Autodesk Inventor part; units mm, degrees
(part 2 of 3)
  line L477 (3.0088, -4.1422) -> (3.0088, -4.3979) construction
  spline S158 degree 3 poles (3.0088, -4.3979) (3.0088, -4.6537) (3.2161, -4.861) (3.4718, -4.861) knots 0 0 0 0 1 1 1 1
  line L478 (3.0088, -4.3979) -> (3.0088, -4.6537) construction
  line L479 (3.0088, -4.6537) -> (3.2161, -4.861) construction
  line L480 (3.2161, -4.861) -> (3.4718, -4.861) construction
  spline S159 degree 3 poles (3.4718, -4.861) (3.7274, -4.861) (3.9348, -4.6537) (3.9348, -4.3979) knots 0 0 0 0 1 1 1 1
  line L481 (3.4718, -4.861) -> (3.7274, -4.861) construction
  line L482 (3.7274, -4.861) -> (3.9348, -4.6537) construction
  line L483 (3.9348, -4.6537) -> (3.9348, -4.3979) construction
  spline S160 degree 3 poles (6.5807, -4.3979) (6.5807, -4.1422) (6.3733, -3.9349) (6.1176, -3.9349) knots 0 0 0 0 1 1 1 1
  line L484 (6.5807, -4.3979) -> (6.5807, -4.1422) construction
  line L485 (6.5807, -4.1422) -> (6.3733, -3.9349) construction
  line L486 (6.3733, -3.9349) -> (6.1176, -3.9349) construction
  spline S161 degree 3 poles (6.1176, -3.9349) (5.862, -3.9349) (5.6547, -4.1422) (5.6547, -4.3979) knots 0 0 0 0 1 1 1 1
  line L487 (6.1176, -3.9349) -> (5.862, -3.9349) construction
  line L488 (5.862, -3.9349) -> (5.6547, -4.1422) construction
  line L489 (5.6547, -4.1422) -> (5.6547, -4.3979) construction
  spline S162 degree 3 poles (5.6547, -4.3979) (5.6547, -4.6537) (5.862, -4.861) (6.1176, -4.861) knots 0 0 0 0 1 1 1 1
  line L490 (5.6547, -4.3979) -> (5.6547, -4.6537) construction
  line L491 (5.6547, -4.6537) -> (5.862, -4.861) construction
  line L492 (5.862, -4.861) -> (6.1176, -4.861) construction
  spline S163 degree 3 poles (6.1176, -4.861) (6.3733, -4.861) (6.5807, -4.6537) (6.5807, -4.3979) knots 0 0 0 0 1 1 1 1
  line L493 (6.1176, -4.861) -> (6.3733, -4.861) construction
  line L494 (6.3733, -4.861) -> (6.5807, -4.6537) construction
  line L495 (6.5807, -4.6537) -> (6.5807, -4.3979) construction
  spline S164 degree 3 poles (9.2265, -4.3979) (9.2265, -4.1422) (9.0191, -3.9349) (8.7634, -3.9349) knots 0 0 0 0 1 1 1 1
  line L496 (9.2265, -4.3979) -> (9.2265, -4.1422) construction
  line L497 (9.2265, -4.1422) -> (9.0191, -3.9349) construction
  line L498 (9.0191, -3.9349) -> (8.7634, -3.9349) construction
  spline S165 degree 3 poles (8.7634, -3.9349) (8.5078, -3.9349) (8.3005, -4.1422) (8.3005, -4.3979) knots 0 0 0 0 1 1 1 1
  line L499 (8.7634, -3.9349) -> (8.5078, -3.9349) construction
  line L500 (8.5078, -3.9349) -> (8.3005, -4.1422) construction
  line L501 (8.3005, -4.1422) -> (8.3005, -4.3979) construction
  spline S166 degree 3 poles (8.3005, -4.3979) (8.3005, -4.6537) (8.5078, -4.861) (8.7634, -4.861) knots 0 0 0 0 1 1 1 1
  line L502 (8.3005, -4.3979) -> (8.3005, -4.6537) construction
  line L503 (8.3005, -4.6537) -> (8.5078, -4.861) construction
  line L504 (8.5078, -4.861) -> (8.7634, -4.861) construction
  spline S167 degree 3 poles (8.7634, -4.861) (9.0191, -4.861) (9.2265, -4.6537) (9.2265, -4.3979) knots 0 0 0 0 1 1 1 1
  line L505 (8.7634, -4.861) -> (9.0191, -4.861) construction
  line L506 (9.0191, -4.861) -> (9.2265, -4.6537) construction
  line L507 (9.2265, -4.6537) -> (9.2265, -4.3979) construction
  spline S168 degree 3 poles (11.8723, -4.3979) (11.8723, -4.1422) (11.6649, -3.9349) (11.4092, -3.9349) knots 0 0 0 0 1 1 1 1
  line L508 (11.8723, -4.3979) -> (11.8723, -4.1422) construction
  line L509 (11.8723, -4.1422) -> (11.6649, -3.9349) construction
  line L510 (11.6649, -3.9349) -> (11.4092, -3.9349) construction
  spline S169 degree 3 poles (11.4092, -3.9349) (11.1536, -3.9349) (10.9463, -4.1422) (10.9463, -4.3979) knots 0 0 0 0 1 1 1 1
  line L511 (11.4092, -3.9349) -> (11.1536, -3.9349) construction
  line L512 (11.1536, -3.9349) -> (10.9463, -4.1422) construction
  line L513 (10.9463, -4.1422) -> (10.9463, -4.3979) construction
  spline S170 degree 3 poles (10.9463, -4.3979) (10.9463, -4.6537) (11.1536, -4.861) (11.4092, -4.861) knots 0 0 0 0 1 1 1 1
  line L514 (10.9463, -4.3979) -> (10.9463, -4.6537) construction
  line L515 (10.9463, -4.6537) -> (11.1536, -4.861) construction
  line L516 (11.1536, -4.861) -> (11.4092, -4.861) construction
  spline S171 degree 3 poles (11.4092, -4.861) (11.6649, -4.861) (11.8723, -4.6537) (11.8723, -4.3979) knots 0 0 0 0 1 1 1 1
  line L517 (11.4092, -4.861) -> (11.6649, -4.861) construction
  line L518 (11.6649, -4.861) -> (11.8723, -4.6537) construction
  line L519 (11.8723, -4.6537) -> (11.8723, -4.3979) construction
  spline S172 degree 3 poles (6.5807, 12.2708) (6.5807, 12.5264) (6.3733, 12.7338) (6.1176, 12.7338) knots 0 0 0 0 1 1 1 1
  line L520 (6.5807, 12.2708) -> (6.5807, 12.5264) construction
  line L521 (6.5807, 12.5264) -> (6.3733, 12.7338) construction
  line L522 (6.3733, 12.7338) -> (6.1176, 12.7338) construction
  spline S173 degree 3 poles (6.1176, 12.7338) (5.862, 12.7338) (5.6547, 12.5264) (5.6547, 12.2708) knots 0 0 0 0 1 1 1 1
  line L523 (6.1176, 12.7338) -> (5.862, 12.7338) construction
  line L524 (5.862, 12.7338) -> (5.6547, 12.5264) construction
  line L525 (5.6547, 12.5264) -> (5.6547, 12.2708) construction
  spline S174 degree 3 poles (5.6547, 12.2708) (5.6547, 12.0151) (5.862, 11.8077) (6.1176, 11.8077) knots 0 0 0 0 1 1 1 1
  line L526 (5.6547, 12.2708) -> (5.6547, 12.0151) construction
  line L527 (5.6547, 12.0151) -> (5.862, 11.8077) construction
  line L528 (5.862, 11.8077) -> (6.1176, 11.8077) construction
  spline S175 degree 3 poles (6.1176, 11.8077) (6.3733, 11.8077) (6.5807, 12.0151) (6.5807, 12.2708) knots 0 0 0 0 1 1 1 1
  line L529 (6.1176, 11.8077) -> (6.3733, 11.8077) construction
  line L530 (6.3733, 11.8077) -> (6.5807, 12.0151) construction
  line L531 (6.5807, 12.0151) -> (6.5807, 12.2708) construction
  spline S176 degree 3 poles (9.2265, 12.2708) (9.2265, 12.5264) (9.0191, 12.7338) (8.7634, 12.7338) knots 0 0 0 0 1 1 1 1
  line L532 (9.2265, 12.2708) -> (9.2265, 12.5264) construction
  line L533 (9.2265, 12.5264) -> (9.0191, 12.7338) construction
  line L534 (9.0191, 12.7338) -> (8.7634, 12.7338) construction
  spline S177 degree 3 poles (8.7634, 12.7338) (8.5078, 12.7338) (8.3005, 12.5264) (8.3005, 12.2708) knots 0 0 0 0 1 1 1 1
  line L535 (8.7634, 12.7338) -> (8.5078, 12.7338) construction
  line L536 (8.5078, 12.7338) -> (8.3005, 12.5264) construction
  line L537 (8.3005, 12.5264) -> (8.3005, 12.2708) construction
  spline S178 degree 3 poles (8.3005, 12.2708) (8.3005, 12.0151) (8.5078, 11.8077) (8.7634, 11.8077) knots 0 0 0 0 1 1 1 1
  line L538 (8.3005, 12.2708) -> (8.3005, 12.0151) construction
  line L539 (8.3005, 12.0151) -> (8.5078, 11.8077) construction
  line L540 (8.5078, 11.8077) -> (8.7634, 11.8077) construction
  spline S179 degree 3 poles (8.7634, 11.8077) (9.0191, 11.8077) (9.2265, 12.0151) (9.2265, 12.2708) knots 0 0 0 0 1 1 1 1
  line L541 (8.7634, 11.8077) -> (9.0191, 11.8077) construction
  line L542 (9.0191, 11.8077) -> (9.2265, 12.0151) construction
  line L543 (9.2265, 12.0151) -> (9.2265, 12.2708) construction
  spline S180 degree 3 poles (9.2265, 17.5624) (9.2265, 17.8181) (9.0191, 18.0255) (8.7634, 18.0255) knots 0 0 0 0 1 1 1 1
  line L544 (9.2265, 17.5624) -> (9.2265, 17.8181) construction
  line L545 (9.2265, 17.8181) -> (9.0191, 18.0255) construction
  line L546 (9.0191, 18.0255) -> (8.7634, 18.0255) construction
  spline S181 degree 3 poles (8.7634, 18.0255) (8.5078, 18.0255) (8.3005, 17.8181) (8.3005, 17.5624) knots 0 0 0 0 1 1 1 1
  line L547 (8.7634, 18.0255) -> (8.5078, 18.0255) construction
  line L548 (8.5078, 18.0255) -> (8.3005, 17.8181) construction
  line L549 (8.3005, 17.8181) -> (8.3005, 17.5624) construction
  spline S182 degree 3 poles (8.3005, 17.5624) (8.3005, 17.3068) (8.5078, 17.0993) (8.7634, 17.0993) knots 0 0 0 0 1 1 1 1
  line L550 (8.3005, 17.5624) -> (8.3005, 17.3068) construction
  line L551 (8.3005, 17.3068) -> (8.5078, 17.0993) construction
  line L552 (8.5078, 17.0993) -> (8.7634, 17.0993) construction
  spline S183 degree 3 poles (8.7634, 17.0993) (9.0191, 17.0993) (9.2265, 17.3068) (9.2265, 17.5624) knots 0 0 0 0 1 1 1 1
  line L553 (8.7634, 17.0993) -> (9.0191, 17.0993) construction
  line L554 (9.0191, 17.0993) -> (9.2265, 17.3068) construction
  line L555 (9.2265, 17.3068) -> (9.2265, 17.5624) construction
  spline S184 degree 3 poles (6.5807, 17.5624) (6.5807, 17.8181) (6.3733, 18.0255) (6.1176, 18.0255) knots 0 0 0 0 1 1 1 1
  line L556 (6.5807, 17.5624) -> (6.5807, 17.8181) construction
  line L557 (6.5807, 17.8181) -> (6.3733, 18.0255) construction
  line L558 (6.3733, 18.0255) -> (6.1176, 18.0255) construction
  spline S185 degree 3 poles (6.1176, 18.0255) (5.862, 18.0255) (5.6547, 17.8181) (5.6547, 17.5624) knots 0 0 0 0 1 1 1 1
  line L559 (6.1176, 18.0255) -> (5.862, 18.0255) construction
  line L560 (5.862, 18.0255) -> (5.6547, 17.8181) construction
  line L561 (5.6547, 17.8181) -> (5.6547, 17.5624) construction
  spline S186 degree 3 poles (5.6547, 17.5624) (5.6547, 17.3068) (5.862, 17.0993) (6.1176, 17.0993) knots 0 0 0 0 1 1 1 1
  line L562 (5.6547, 17.5624) -> (5.6547, 17.3068) construction
  line L563 (5.6547, 17.3068) -> (5.862, 17.0993) construction
  line L564 (5.862, 17.0993) -> (6.1176, 17.0993) construction
  spline S187 degree 3 poles (6.1176, 17.0993) (6.3733, 17.0993) (6.5807, 17.3068) (6.5807, 17.5624) knots 0 0 0 0 1 1 1 1
  line L565 (6.1176, 17.0993) -> (6.3733, 17.0993) construction
  line L566 (6.3733, 17.0993) -> (6.5807, 17.3068) construction
  line L567 (6.5807, 17.3068) -> (6.5807, 17.5624) construction
  spline S188 degree 3 poles (6.5807, 14.9166) (6.5807, 15.1723) (6.3733, 15.3797) (6.1176, 15.3797) knots 0 0 0 0 1 1 1 1
  line L568 (6.5807, 14.9166) -> (6.5807, 15.1723) construction
  line L569 (6.5807, 15.1723) -> (6.3733, 15.3797) construction
  line L570 (6.3733, 15.3797) -> (6.1176, 15.3797) construction
  spline S189 degree 3 poles (6.1176, 15.3797) (5.862, 15.3797) (5.6547, 15.1723) (5.6547, 14.9166) knots 0 0 0 0 1 1 1 1
  line L571 (6.1176, 15.3797) -> (5.862, 15.3797) construction
  line L572 (5.862, 15.3797) -> (5.6547, 15.1723) construction
  line L573 (5.6547, 15.1723) -> (5.6547, 14.9166) construction
  spline S190 degree 3 poles (5.6547, 14.9166) (5.6547, 14.661) (5.862, 14.4535) (6.1176, 14.4535) knots 0 0 0 0 1 1 1 1
  line L574 (5.6547, 14.9166) -> (5.6547, 14.661) construction
  line L575 (5.6547, 14.661) -> (5.862, 14.4535) construction
  line L576 (5.862, 14.4535) -> (6.1176, 14.4535) construction
  spline S191 degree 3 poles (6.1176, 14.4535) (6.3733, 14.4535) (6.5807, 14.661) (6.5807, 14.9166) knots 0 0 0 0 1 1 1 1
  line L577 (6.1176, 14.4535) -> (6.3733, 14.4535) construction
  line L578 (6.3733, 14.4535) -> (6.5807, 14.661) construction
  line L579 (6.5807, 14.661) -> (6.5807, 14.9166) construction
  spline S192 degree 3 poles (9.2265, 14.9166) (9.2265, 15.1723) (9.0191, 15.3797) (8.7634, 15.3797) knots 0 0 0 0 1 1 1 1
  line L580 (9.2265, 14.9166) -> (9.2265, 15.1723) construction
  line L581 (9.2265, 15.1723) -> (9.0191, 15.3797) construction
  line L582 (9.0191, 15.3797) -> (8.7634, 15.3797) construction
  spline S193 degree 3 poles (8.7634, 15.3797) (8.5078, 15.3797) (8.3005, 15.1723) (8.3005, 14.9166) knots 0 0 0 0 1 1 1 1
  line L583 (8.7634, 15.3797) -> (8.5078, 15.3797) construction
  line L584 (8.5078, 15.3797) -> (8.3005, 15.1723) construction
  line L585 (8.3005, 15.1723) -> (8.3005, 14.9166) construction
  spline S194 degree 3 poles (8.3005, 14.9166) (8.3005, 14.661) (8.5078, 14.4535) (8.7634, 14.4535) knots 0 0 0 0 1 1 1 1
  line L586 (8.3005, 14.9166) -> (8.3005, 14.661) construction
  line L587 (8.3005, 14.661) -> (8.5078, 14.4535) construction
  line L588 (8.5078, 14.4535) -> (8.7634, 14.4535) construction
  spline S195 degree 3 poles (8.7634, 14.4535) (9.0191, 14.4535) (9.2265, 14.661) (9.2265, 14.9166) knots 0 0 0 0 1 1 1 1
  line L589 (8.7634, 14.4535) -> (9.0191, 14.4535) construction
  line L590 (9.0191, 14.4535) -> (9.2265, 14.661) construction
  line L591 (9.2265, 14.661) -> (9.2265, 14.9166) construction
  spline S196 degree 3 poles (6.5807, 1.6875) (6.5807, 1.9432) (6.3733, 2.1506) (6.1176, 2.1506) knots 0 0 0 0 1 1 1 1
  line L592 (6.5807, 1.6875) -> (6.5807, 1.9432) construction
  line L593 (6.5807, 1.9432) -> (6.3733, 2.1506) construction
  line L594 (6.3733, 2.1506) -> (6.1176, 2.1506) construction
  spline S197 degree 3 poles (6.1176, 2.1506) (5.862, 2.1506) (5.6547, 1.9432) (5.6547, 1.6875) knots 0 0 0 0 1 1 1 1
  line L595 (6.1176, 2.1506) -> (5.862, 2.1506) construction
  line L596 (5.862, 2.1506) -> (5.6547, 1.9432) construction
  line L597 (5.6547, 1.9432) -> (5.6547, 1.6875) construction
  spline S198 degree 3 poles (5.6547, 1.6875) (5.6547, 1.4319) (5.862, 1.2244) (6.1176, 1.2244) knots 0 0 0 0 1 1 1 1
  line L598 (5.6547, 1.6875) -> (5.6547, 1.4319) construction
  line L599 (5.6547, 1.4319) -> (5.862, 1.2244) construction
  line L600 (5.862, 1.2244) -> (6.1176, 1.2244) construction
  spline S199 degree 3 poles (6.1176, 1.2244) (6.3733, 1.2244) (6.5807, 1.4319) (6.5807, 1.6875) knots 0 0 0 0 1 1 1 1
  line L601 (6.1176, 1.2244) -> (6.3733, 1.2244) construction
  line L602 (6.3733, 1.2244) -> (6.5807, 1.4319) construction
  line L603 (6.5807, 1.4319) -> (6.5807, 1.6875) construction
  spline S200 degree 3 poles (9.2265, 1.6875) (9.2265, 1.9432) (9.0191, 2.1506) (8.7634, 2.1506) knots 0 0 0 0 1 1 1 1
  line L604 (9.2265, 1.6875) -> (9.2265, 1.9432) construction
  line L605 (9.2265, 1.9432) -> (9.0191, 2.1506) construction
  line L606 (9.0191, 2.1506) -> (8.7634, 2.1506) construction
  spline S201 degree 3 poles (8.7634, 2.1506) (8.5078, 2.1506) (8.3005, 1.9432) (8.3005, 1.6875) knots 0 0 0 0 1 1 1 1
  line L607 (8.7634, 2.1506) -> (8.5078, 2.1506) construction
  line L608 (8.5078, 2.1506) -> (8.3005, 1.9432) construction
  line L609 (8.3005, 1.9432) -> (8.3005, 1.6875) construction
  spline S202 degree 3 poles (8.3005, 1.6875) (8.3005, 1.4319) (8.5078, 1.2244) (8.7634, 1.2244) knots 0 0 0 0 1 1 1 1
  line L610 (8.3005, 1.6875) -> (8.3005, 1.4319) construction
  line L611 (8.3005, 1.4319) -> (8.5078, 1.2244) construction
  line L612 (8.5078, 1.2244) -> (8.7634, 1.2244) construction
  spline S203 degree 3 poles (8.7634, 1.2244) (9.0191, 1.2244) (9.2265, 1.4319) (9.2265, 1.6875) knots 0 0 0 0 1 1 1 1
  line L613 (8.7634, 1.2244) -> (9.0191, 1.2244) construction
  line L614 (9.0191, 1.2244) -> (9.2265, 1.4319) construction
  line L615 (9.2265, 1.4319) -> (9.2265, 1.6875) construction
  spline S204 degree 3 poles (6.5807, 30.7915) (6.5807, 31.0472) (6.3733, 31.2546) (6.1176, 31.2546) knots 0 0 0 0 1 1 1 1
  line L616 (6.5807, 30.7915) -> (6.5807, 31.0472) construction
  line L617 (6.5807, 31.0472) -> (6.3733, 31.2546) construction
  line L618 (6.3733, 31.2546) -> (6.1176, 31.2546) construction
  spline S205 degree 3 poles (6.1176, 31.2546) (5.862, 31.2546) (5.6547, 31.0472) (5.6547, 30.7915) knots 0 0 0 0 1 1 1 1
  line L619 (6.1176, 31.2546) -> (5.862, 31.2546) construction
  line L620 (5.862, 31.2546) -> (5.6547, 31.0472) construction
  line L621 (5.6547, 31.0472) -> (5.6547, 30.7915) construction
  spline S206 degree 3 poles (5.6547, 30.7915) (5.6547, 30.5359) (5.862, 30.3284) (6.1176, 30.3284) knots 0 0 0 0 1 1 1 1
  line L622 (5.6547, 30.7915) -> (5.6547, 30.5359) construction
  line L623 (5.6547, 30.5359) -> (5.862, 30.3284) construction
  line L624 (5.862, 30.3284) -> (6.1176, 30.3284) construction
  spline S207 degree 3 poles (6.1176, 30.3284) (6.3733, 30.3284) (6.5807, 30.5359) (6.5807, 30.7915) knots 0 0 0 0 1 1 1 1
  line L625 (6.1176, 30.3284) -> (6.3733, 30.3284) construction
  line L626 (6.3733, 30.3284) -> (6.5807, 30.5359) construction
  line L627 (6.5807, 30.5359) -> (6.5807, 30.7915) construction
  spline S208 degree 3 poles (9.2265, 30.7915) (9.2265, 31.0472) (9.0191, 31.2546) (8.7634, 31.2546) knots 0 0 0 0 1 1 1 1
  line L628 (9.2265, 30.7915) -> (9.2265, 31.0472) construction
  line L629 (9.2265, 31.0472) -> (9.0191, 31.2546) construction
  line L630 (9.0191, 31.2546) -> (8.7634, 31.2546) construction
  spline S209 degree 3 poles (8.7634, 31.2546) (8.5078, 31.2546) (8.3005, 31.0472) (8.3005, 30.7915) knots 0 0 0 0 1 1 1 1
  line L631 (8.7634, 31.2546) -> (8.5078, 31.2546) construction
  line L632 (8.5078, 31.2546) -> (8.3005, 31.0472) construction
  line L633 (8.3005, 31.0472) -> (8.3005, 30.7915) construction
  spline S210 degree 3 poles (8.3005, 30.7915) (8.3005, 30.5359) (8.5078, 30.3284) (8.7634, 30.3284) knots 0 0 0 0 1 1 1 1
  line L634 (8.3005, 30.7915) -> (8.3005, 30.5359) construction
  line L635 (8.3005, 30.5359) -> (8.5078, 30.3284) construction
  line L636 (8.5078, 30.3284) -> (8.7634, 30.3284) construction
  spline S211 degree 3 poles (8.7634, 30.3284) (9.0191, 30.3284) (9.2265, 30.5359) (9.2265, 30.7915) knots 0 0 0 0 1 1 1 1
  line L637 (8.7634, 30.3284) -> (9.0191, 30.3284) construction
  line L638 (9.0191, 30.3284) -> (9.2265, 30.5359) construction
  line L639 (9.2265, 30.5359) -> (9.2265, 30.7915) construction
  spline S212 degree 3 poles (9.2265, 28.1457) (9.2265, 28.4013) (9.0191, 28.6088) (8.7634, 28.6088) knots 0 0 0 0 1 1 1 1
  line L640 (9.2265, 28.1457) -> (9.2265, 28.4013) construction
  line L641 (9.2265, 28.4013) -> (9.0191, 28.6088) construction
  line L642 (9.0191, 28.6088) -> (8.7634, 28.6088) construction
  spline S213 degree 3 poles (8.7634, 28.6088) (8.5078, 28.6088) (8.3005, 28.4013) (8.3005, 28.1457) knots 0 0 0 0 1 1 1 1
  line L643 (8.7634, 28.6088) -> (8.5078, 28.6088) construction
  line L644 (8.5078, 28.6088) -> (8.3005, 28.4013) construction
  line L645 (8.3005, 28.4013) -> (8.3005, 28.1457) construction
  spline S214 degree 3 poles (8.3005, 28.1457) (8.3005, 27.89) (8.5078, 27.6826) (8.7634, 27.6826) knots 0 0 0 0 1 1 1 1
  line L646 (8.3005, 28.1457) -> (8.3005, 27.89) construction
  line L647 (8.3005, 27.89) -> (8.5078, 27.6826) construction
  line L648 (8.5078, 27.6826) -> (8.7634, 27.6826) construction
  spline S215 degree 3 poles (8.7634, 27.6826) (9.0191, 27.6826) (9.2265, 27.89) (9.2265, 28.1457) knots 0 0 0 0 1 1 1 1
  line L649 (8.7634, 27.6826) -> (9.0191, 27.6826) construction
  line L650 (9.0191, 27.6826) -> (9.2265, 27.89) construction
  line L651 (9.2265, 27.89) -> (9.2265, 28.1457) construction
  spline S216 degree 3 poles (6.5807, 28.1457) (6.5807, 28.4013) (6.3733, 28.6088) (6.1176, 28.6088) knots 0 0 0 0 1 1 1 1
  line L652 (6.5807, 28.1457) -> (6.5807, 28.4013) construction
  line L653 (6.5807, 28.4013) -> (6.3733, 28.6088) construction
  line L654 (6.3733, 28.6088) -> (6.1176, 28.6088) construction
  spline S217 degree 3 poles (6.1176, 28.6088) (5.862, 28.6088) (5.6547, 28.4013) (5.6547, 28.1457) knots 0 0 0 0 1 1 1 1
  line L655 (6.1176, 28.6088) -> (5.862, 28.6088) construction
  line L656 (5.862, 28.6088) -> (5.6547, 28.4013) construction
  line L657 (5.6547, 28.4013) -> (5.6547, 28.1457) construction
  spline S218 degree 3 poles (5.6547, 28.1457) (5.6547, 27.89) (5.862, 27.6826) (6.1176, 27.6826) knots 0 0 0 0 1 1 1 1
  line L658 (5.6547, 28.1457) -> (5.6547, 27.89) construction
  line L659 (5.6547, 27.89) -> (5.862, 27.6826) construction
  line L660 (5.862, 27.6826) -> (6.1176, 27.6826) construction
  spline S219 degree 3 poles (6.1176, 27.6826) (6.3733, 27.6826) (6.5807, 27.89) (6.5807, 28.1457) knots 0 0 0 0 1 1 1 1
  line L661 (6.1176, 27.6826) -> (6.3733, 27.6826) construction
  line L662 (6.3733, 27.6826) -> (6.5807, 27.89) construction
  line L663 (6.5807, 27.89) -> (6.5807, 28.1457) construction
  spline S220 degree 3 poles (6.5807, -0.9584) (6.5807, -0.7026) (6.3733, -0.4954) (6.1176, -0.4954) knots 0 0 0 0 1 1 1 1
  line L664 (6.5807, -0.9584) -> (6.5807, -0.7026) construction
  line L665 (6.5807, -0.7026) -> (6.3733, -0.4954) construction
  line L666 (6.3733, -0.4954) -> (6.1176, -0.4954) construction
  spline S221 degree 3 poles (6.1176, -0.4954) (5.862, -0.4954) (5.6547, -0.7026) (5.6547, -0.9584) knots 0 0 0 0 1 1 1 1
  line L667 (6.1176, -0.4954) -> (5.862, -0.4954) construction
  line L668 (5.862, -0.4954) -> (5.6547, -0.7026) construction
  line L669 (5.6547, -0.7026) -> (5.6547, -0.9584) construction
  spline S222 degree 3 poles (5.6547, -0.9584) (5.6547, -1.2141) (5.862, -1.4214) (6.1176, -1.4214) knots 0 0 0 0 1 1 1 1
  line L670 (5.6547, -0.9584) -> (5.6547, -1.2141) construction
  line L671 (5.6547, -1.2141) -> (5.862, -1.4214) construction
  line L672 (5.862, -1.4214) -> (6.1176, -1.4214) construction
  spline S223 degree 3 poles (6.1176, -1.4214) (6.3733, -1.4214) (6.5807, -1.2141) (6.5807, -0.9584) knots 0 0 0 0 1 1 1 1
  line L673 (6.1176, -1.4214) -> (6.3733, -1.4214) construction
  line L674 (6.3733, -1.4214) -> (6.5807, -1.2141) construction
  line L675 (6.5807, -1.2141) -> (6.5807, -0.9584) construction
  spline S224 degree 3 poles (9.2265, -0.9584) (9.2265, -0.7026) (9.0191, -0.4954) (8.7634, -0.4954) knots 0 0 0 0 1 1 1 1
  line L676 (9.2265, -0.9584) -> (9.2265, -0.7026) construction
  line L677 (9.2265, -0.7026) -> (9.0191, -0.4954) construction
  line L678 (9.0191, -0.4954) -> (8.7634, -0.4954) construction
  spline S225 degree 3 poles (8.7634, -0.4954) (8.5078, -0.4954) (8.3005, -0.7026) (8.3005, -0.9584) knots 0 0 0 0 1 1 1 1
  line L679 (8.7634, -0.4954) -> (8.5078, -0.4954) construction
  line L680 (8.5078, -0.4954) -> (8.3005, -0.7026) construction
  line L681 (8.3005, -0.7026) -> (8.3005, -0.9584) construction
  spline S226 degree 3 poles (8.3005, -0.9584) (8.3005, -1.2141) (8.5078, -1.4214) (8.7634, -1.4214) knots 0 0 0 0 1 1 1 1
  line L682 (8.3005, -0.9584) -> (8.3005, -1.2141) construction
  line L683 (8.3005, -1.2141) -> (8.5078, -1.4214) construction
  line L684 (8.5078, -1.4214) -> (8.7634, -1.4214) construction
  spline S227 degree 3 poles (8.7634, -1.4214) (9.0191, -1.4214) (9.2265, -1.2141) (9.2265, -0.9584) knots 0 0 0 0 1 1 1 1
  line L685 (8.7634, -1.4214) -> (9.0191, -1.4214) construction
  line L686 (9.0191, -1.4214) -> (9.2265, -1.2141) construction
  line L687 (9.2265, -1.2141) -> (9.2265, -0.9584) construction
  spline S228 degree 3 poles (3.9348, -4.3979) (3.9348, -4.1422) (3.7274, -3.9349) (3.4718, -3.9349) knots 0 0 0 0 1 1 1 1
  line L688 (3.9348, -4.3979) -> (3.9348, -4.1422) construction
  line L689 (3.9348, -4.1422) -> (3.7274, -3.9349) construction
  line L690 (3.7274, -3.9349) -> (3.4718, -3.9349) construction
  spline S229 degree 3 poles (3.4718, -3.9349) (3.2161, -3.9349) (3.0088, -4.1422) (3.0088, -4.3979) knots 0 0 0 0 1 1 1 1
  line L691 (3.4718, -3.9349) -> (3.2161, -3.9349) construction
  line L692 (3.2161, -3.9349) -> (3.0088, -4.1422) construction
  line L693 (3.0088, -4.1422) -> (3.0088, -4.3979) construction
  spline S230 degree 3 poles (3.0088, -4.3979) (3.0088, -4.6537) (3.2161, -4.861) (3.4718, -4.861) knots 0 0 0 0 1 1 1 1
  line L694 (3.0088, -4.3979) -> (3.0088, -4.6537) construction
  line L695 (3.0088, -4.6537) -> (3.2161, -4.861) construction
  line L696 (3.2161, -4.861) -> (3.4718, -4.861) construction
  spline S231 degree 3 poles (3.4718, -4.861) (3.7274, -4.861) (3.9348, -4.6537) (3.9348, -4.3979) knots 0 0 0 0 1 1 1 1
  line L697 (3.4718, -4.861) -> (3.7274, -4.861) construction
  line L698 (3.7274, -4.861) -> (3.9348, -4.6537) construction
  line L699 (3.9348, -4.6537) -> (3.9348, -4.3979) construction
  spline S232 degree 3 poles (6.5807, -4.3979) (6.5807, -4.1422) (6.3733, -3.9349) (6.1176, -3.9349) knots 0 0 0 0 1 1 1 1
  line L700 (6.5807, -4.3979) -> (6.5807, -4.1422) construction
  line L701 (6.5807, -4.1422) -> (6.3733, -3.9349) construction
  line L702 (6.3733, -3.9349) -> (6.1176, -3.9349) construction
  spline S233 degree 3 poles (6.1176, -3.9349) (5.862, -3.9349) (5.6547, -4.1422) (5.6547, -4.3979) knots 0 0 0 0 1 1 1 1
  line L703 (6.1176, -3.9349) -> (5.862, -3.9349) construction
  line L704 (5.862, -3.9349) -> (5.6547, -4.1422) construction
  line L705 (5.6547, -4.1422) -> (5.6547, -4.3979) construction
  spline S234 degree 3 poles (5.6547, -4.3979) (5.6547, -4.6537) (5.862, -4.861) (6.1176, -4.861) knots 0 0 0 0 1 1 1 1
  line L706 (5.6547, -4.3979) -> (5.6547, -4.6537) construction
  line L707 (5.6547, -4.6537) -> (5.862, -4.861) construction
  line L708 (5.862, -4.861) -> (6.1176, -4.861) construction
  spline S235 degree 3 poles (6.1176, -4.861) (6.3733, -4.861) (6.5807, -4.6537) (6.5807, -4.3979) knots 0 0 0 0 1 1 1 1
  line L709 (6.1176, -4.861) -> (6.3733, -4.861) construction
  line L710 (6.3733, -4.861) -> (6.5807, -4.6537) construction
  line L711 (6.5807, -4.6537) -> (6.5807, -4.3979) construction
  spline S236 degree 3 poles (9.2265, -4.3979) (9.2265, -4.1422) (9.0191, -3.9349) (8.7634, -3.9349) knots 0 0 0 0 1 1 1 1
  line L712 (9.2265, -4.3979) -> (9.2265, -4.1422) construction
  line L713 (9.2265, -4.1422) -> (9.0191, -3.9349) construction
  line L714 (9.0191, -3.9349) -> (8.7634, -3.9349) construction
  spline S237 degree 3 poles (8.7634, -3.9349) (8.5078, -3.9349) (8.3005, -4.1422) (8.3005, -4.3979) knots 0 0 0 0 1 1 1 1
  line L715 (8.7634, -3.9349) -> (8.5078, -3.9349) construction
  line L716 (8.5078, -3.9349) -> (8.3005, -4.1422) construction
  line L717 (8.3005, -4.1422) -> (8.3005, -4.3979) construction
  spline S238 degree 3 poles (8.3005, -4.3979) (8.3005, -4.6537) (8.5078, -4.861) (8.7634, -4.861) knots 0 0 0 0 1 1 1 1
  line L718 (8.3005, -4.3979) -> (8.3005, -4.6537) construction
  line L719 (8.3005, -4.6537) -> (8.5078, -4.861) construction
  line L720 (8.5078, -4.861) -> (8.7634, -4.861) construction
  spline S239 degree 3 poles (8.7634, -4.861) (9.0191, -4.861) (9.2265, -4.6537) (9.2265, -4.3979) knots 0 0 0 0 1 1 1 1
  line L721 (8.7634, -4.861) -> (9.0191, -4.861) construction
  line L722 (9.0191, -4.861) -> (9.2265, -4.6537) construction
  line L723 (9.2265, -4.6537) -> (9.2265, -4.3979) construction
  spline S240 degree 3 poles (11.8723, -4.3979) (11.8723, -4.1422) (11.6649, -3.9349) (11.4092, -3.9349) knots 0 0 0 0 1 1 1 1
  line L724 (11.8723, -4.3979) -> (11.8723, -4.1422) construction
  line L725 (11.8723, -4.1422) -> (11.6649, -3.9349) construction
  line L726 (11.6649, -3.9349) -> (11.4092, -3.9349) construction
  spline S241 degree 3 poles (11.4092, -3.9349) (11.1536, -3.9349) (10.9463, -4.1422) (10.9463, -4.3979) knots 0 0 0 0 1 1 1 1
  line L727 (11.4092, -3.9349) -> (11.1536, -3.9349) construction
  line L728 (11.1536, -3.9349) -> (10.9463, -4.1422) construction
  line L729 (10.9463, -4.1422) -> (10.9463, -4.3979) construction
  spline S242 degree 3 poles (10.9463, -4.3979) (10.9463, -4.6537) (11.1536, -4.861) (11.4092, -4.861) knots 0 0 0 0 1 1 1 1
  line L730 (10.9463, -4.3979) -> (10.9463, -4.6537) construction
  line L731 (10.9463, -4.6537) -> (11.1536, -4.861) construction
  line L732 (11.1536, -4.861) -> (11.4092, -4.861) construction
  spline S243 degree 3 poles (11.4092, -4.861) (11.6649, -4.861) (11.8723, -4.6537) (11.8723, -4.3979) knots 0 0 0 0 1 1 1 1
  line L733 (11.4092, -4.861) -> (11.6649, -4.861) construction
  line L734 (11.6649, -4.861) -> (11.8723, -4.6537) construction
  line L735 (11.8723, -4.6537) -> (11.8723, -4.3979) construction
  spline S244 degree 3 poles (3.6041, 14.9166) (3.6041, 15.574) (3.071, 16.1072) (2.4136, 16.1072) knots 0 0 0 0 1 1 1 1
  line L736 (3.6041, 14.9166) -> (3.6041, 15.574) construction
  line L737 (3.6041, 15.574) -> (3.071, 16.1072) construction
  line L738 (3.071, 16.1072) -> (2.4136, 16.1072) construction
  spline S245 degree 3 poles (2.4136, 16.1072) (1.7561, 16.1072) (1.2229, 15.574) (1.2229, 14.9166) knots 0 0 0 0 1 1 1 1
  line L739 (2.4136, 16.1072) -> (1.7561, 16.1072) construction
  line L740 (1.7561, 16.1072) -> (1.2229, 15.574) construction
  line L741 (1.2229, 15.574) -> (1.2229, 14.9166) construction
  spline S246 degree 3 poles (1.2229, 14.9166) (1.2229, 14.2592) (1.7561, 13.726) (2.4136, 13.726) knots 0 0 0 0 1 1 1 1
  line L742 (1.2229, 14.9166) -> (1.2229, 14.2592) construction
  line L743 (1.2229, 14.2592) -> (1.7561, 13.726) construction
  line L744 (1.7561, 13.726) -> (2.4136, 13.726) construction
  spline S247 degree 3 poles (2.4136, 13.726) (3.071, 13.726) (3.6041, 14.2592) (3.6041, 14.9166) knots 0 0 0 0 1 1 1 1
  line L745 (2.4136, 13.726) -> (3.071, 13.726) construction
  line L746 (3.071, 13.726) -> (3.6041, 14.2592) construction
  line L747 (3.6041, 14.2592) -> (3.6041, 14.9166) construction
  spline S248 degree 3 poles (13.6583, 14.9166) (13.6583, 15.574) (13.125, 16.1072) (12.4676, 16.1072) knots 0 0 0 0 1 1 1 1
  line L748 (13.6583, 14.9166) -> (13.6583, 15.574) construction
  line L749 (13.6583, 15.574) -> (13.125, 16.1072) construction
  line L750 (13.125, 16.1072) -> (12.4676, 16.1072) construction
  spline S249 degree 3 poles (12.4676, 16.1072) (11.8102, 16.1072) (11.277, 15.574) (11.277, 14.9166) knots 0 0 0 0 1 1 1 1
  line L751 (12.4676, 16.1072) -> (11.8102, 16.1072) construction
  line L752 (11.8102, 16.1072) -> (11.277, 15.574) construction
  line L753 (11.277, 15.574) -> (11.277, 14.9166) construction
  spline S250 degree 3 poles (11.277, 14.9166) (11.277, 14.2592) (11.8102, 13.726) (12.4676, 13.726) knots 0 0 0 0 1 1 1 1
  line L754 (11.277, 14.9166) -> (11.277, 14.2592) construction
  line L755 (11.277, 14.2592) -> (11.8102, 13.726) construction
  line L756 (11.8102, 13.726) -> (12.4676, 13.726) construction
  spline S251 degree 3 poles (12.4676, 13.726) (13.125, 13.726) (13.6583, 14.2592) (13.6583, 14.9166) knots 0 0 0 0 1 1 1 1
  line L757 (12.4676, 13.726) -> (13.125, 13.726) construction
  line L758 (13.125, 13.726) -> (13.6583, 14.2592) construction
  line L759 (13.6583, 14.2592) -> (13.6583, 14.9166) construction
  spline S252 degree 3 poles (8.6312, 33.9664) (8.6312, 34.6239) (8.0979, 35.1571) (7.4405, 35.1571) knots 0 0 0 0 1 1 1 1
  line L760 (8.6312, 33.9664) -> (8.6312, 34.6239) construction
  line L761 (8.6312, 34.6239) -> (8.0979, 35.1571) construction
  line L762 (8.0979, 35.1571) -> (7.4405, 35.1571) construction
  spline S253 degree 3 poles (7.4405, 35.1571) (6.7831, 35.1571) (6.2499, 34.6239) (6.2499, 33.9664) knots 0 0 0 0 1 1 1 1
  line L763 (7.4405, 35.1571) -> (6.7831, 35.1571) construction
  line L764 (6.7831, 35.1571) -> (6.2499, 34.6239) construction
  line L765 (6.2499, 34.6239) -> (6.2499, 33.9664) construction
  spline S254 degree 3 poles (6.2499, 33.9664) (6.2499, 33.309) (6.7831, 32.7759) (7.4405, 32.7759) knots 0 0 0 0 1 1 1 1
  line L766 (6.2499, 33.9664) -> (6.2499, 33.309) construction
  line L767 (6.2499, 33.309) -> (6.7831, 32.7759) construction
  line L768 (6.7831, 32.7759) -> (7.4405, 32.7759) construction
  spline S255 degree 3 poles (7.4405, 32.7759) (8.0979, 32.7759) (8.6312, 33.309) (8.6312, 33.9664) knots 0 0 0 0 1 1 1 1
  line L769 (7.4405, 32.7759) -> (8.0979, 32.7759) construction
  line L770 (8.0979, 32.7759) -> (8.6312, 33.309) construction
  line L771 (8.6312, 33.309) -> (8.6312, 33.9664) construction
  line L772 (6.1176, 28.4102) -> (6.1176, 28.1457)
  line L773 (7.4405, 35.1571) -> (7.4405, 32.7759)
  line L774 (6.2499, 33.9664) -> (8.6312, 33.9664)
  circle A0 centre (7.4406, 33.9664) radius 1.1907
  line L775 (2.4136, 16.1072) -> (2.4136, 13.726)
  line L776 (1.2229, 14.9166) -> (3.6041, 14.9166)
  circle A1 centre (2.4135, 14.9166) radius 1.1905
  line L777 (12.4676, 16.1072) -> (12.4676, 13.726)
  line L778 (11.277, 14.9166) -> (13.6583, 14.9166)
  circle A2 centre (12.4677, 14.9166) radius 1.1905
  point P0 (0, 0)
  dimension "d1" = 6.35
  constraints: 22 end point, 5 perpendicular, 3 midpoint, 1 parallel, 777 other
  measures "d1" distance of L2.start L2.end
sketch "Sketch2" plane through (0, 0, 0) normal (0, 1, 0) x (-1, 0, 0)
  line L0 (3.2572, 21.0343) -> (-3.2024, 21.0343)
  line L1 (7.1163, 17.064) -> (7.1163, -17.0656)
  line L2 (-7.1712, 17.0656) -> (-7.1712, -17.0334)
  line L3 (-3.2023, -21.0343) -> (3.1476, -21.0343)
  circle A0 centre (-0.0274, 18.9176) radius 1.1907
  circle A1 centre (-5.0545, -0.1323) radius 1.1905
  circle A2 centre (4.9996, -0.1323) radius 1.1905
  arc A3 (7.1163, 17.064) -> (3.2572, 21.0343) centre (3.2572, 17.1737) ccw
  arc A4 (-3.2024, 21.0343) -> (-7.1712, 17.0656) centre (-3.2024, 17.0656) ccw
  arc A5 (-7.1712, -17.0334) -> (-3.2023, -21.0343) centre (-3.1701, -17.0334) ccw
  arc A6 (3.1476, -21.0343) -> (7.1163, -17.0656) centre (3.1476, -17.0656) ccw
  line L4 (-7.1712, 0.0161) -> (7.1163, -0.0008) construction
  line L5 (0.0274, 21.0343) -> (-0.0274, -21.0343) construction
  line L6 (7.2163, -17.0656) -> (7.2163, 17.0626)
  arc A7 (7.2163, 17.0626) -> (3.2572, 21.1343) centre (3.2572, 17.1737) ccw
  line L7 (3.2572, 21.1343) -> (-3.2024, 21.1343)
  arc A8 (-3.2024, 21.1343) -> (-7.2712, 17.0656) centre (-3.2024, 17.0656) ccw
  line L8 (-7.2712, 17.0656) -> (-7.2712, -17.0334)
  arc A9 (-7.2712, -17.0334) -> (-3.2027, -21.1343) centre (-3.1701, -17.0334) ccw
  line L9 (-3.2027, -21.1343) -> (3.1476, -21.1343)
  arc A10 (3.1476, -21.1343) -> (7.2163, -17.0656) centre (3.1476, -17.0656) ccw
  line L10 (9.2163, 17.0374) -> (9.2163, -17.0656)
  arc A11 (3.1476, -23.1343) -> (9.2163, -17.0656) centre (3.1476, -17.0656) ccw
  line L11 (3.1476, -23.1343) -> (-3.2099, -23.1343)
  arc A12 (-9.2712, -17.0334) -> (-3.2099, -23.1343) centre (-3.1701, -17.0334) ccw
  line L12 (-9.2712, -17.0334) -> (-9.2712, 17.0656)
  arc A13 (-3.2024, 23.1343) -> (-9.2712, 17.0656) centre (-3.2024, 17.0656) ccw
  line L13 (-3.2024, 23.1343) -> (3.2572, 23.1343)
  arc A14 (9.2163, 17.0374) -> (3.2572, 23.1343) centre (3.2572, 17.1737) ccw
  circle A15 centre (-0.0274, 18.9176) radius 1.7907
  arc A16 (-3.1025, 21.1343) -> (3.0476, 21.1343) centre (-0.0274, 18.9176) ccw
  circle A17 centre (-5.0545, -0.1323) radius 1.7905
  arc A18 (-7.2712, -3.2071) -> (-7.2712, 2.9426) centre (-5.0545, -0.1323) ccw
  circle A19 centre (4.9996, -0.1323) radius 1.7905
  arc A20 (7.2163, 2.9426) -> (7.2163, -3.2071) centre (4.9996, -0.1323) ccw
  arc A21 (-7.2712, 2.9426) -> (-7.2712, -3.2071) centre (-5.0545, -0.1323) ccw
  arc A22 (7.2163, -3.2071) -> (7.2163, 2.9426) centre (4.9996, -0.1323) ccw
  arc A23 (3.0476, 21.1343) -> (-3.1025, 21.1343) centre (-0.0274, 18.9176) ccw
  line L14 (-5.0545, -16.0917) -> (-5.0545, -27.1342)
  line L15 (4.9996, -16.0917) -> (4.9996, -27.1342)
  point P0 (0, 0)
  point P1 (0, 0)
  point P2 (6.0256, 19.8645)
  dimension "d2" = 0.1
  dimension "d3" = 2
  dimension "d4" = 0.6
  dimension "d5" = 2
  dimension "d6" = 0.6
  dimension "d7" = 2
  dimension "d8" = 0.6
  dimension "d9" = 2
  constraints: 37 point on circle, 32 end point, 24 centre point, 6 coincident, 6 point on line, 6 tangent, 5 midpoint, 2 horizontal, 2 vertical, 1 parallel, 1 perpendicular, 21 other
  measures "d2" distance between parallel lines of L2 L8
  measures "d3" distance between parallel lines of L12 L8
  measures "d4" radial gap between concentric circles of A0 A15
  measures "d5" radial gap between concentric circles of A15 A16
  measures "d6" radial gap between concentric circles of A1 A17
  measures "d7" radial gap between concentric circles of A17 A18
  measures "d8" radial gap between concentric circles of A2 A19
  measures "d9" radial gap between concentric circles of A19 A20
extrude "Extrusion1" add sketch "Sketch2" along normal blind 1.5 contours A3 L1 A20 A6 L3 A5 L2 A18 A4 L0 A16 | L0 A16 L7 A7 L6 A20 L1 A3 | A16 L0 | L0 A16 L7 | L0 A4 L2 A18 L8 A8 L7 A16 | A23 L7 A8 L8 A21 A9 L14 A12 L12 A13 L13 A14 L10 A11 L15 A10 L6 A22 A7 | L7 A23 | A20 L6 L1 | L1 A20 | A20 L6 A10 L15 A6 L1 | A22 L6 | A18 L2 | L2 A18 L8 | L15 A10 L9 A9 L14 A5 L3 A6 | L2 A5 L14 A9 L8 A18 | L8 A21 | L15 A11 L11 A12 L14 A9 L9 A10 | A0 | A1 | A2 | A15 | A17 | A19
extrude "Extrusion2" cut sketch "Sketch2" along normal blind 1.5 contours A0 | A1 | A2 | A15 | A17 | A19
extrude "Extrusion4" add sketch "Sketch2" along normal blind 5 contours A23 L7 A8 L8 A21 A9 L14 A12 L12 A13 L13 A14 L10 A11 L15 A10 L6 A22 A7 | L7 A23 | A22 L6 | L8 A21 | L15 A11 L11 A12 L14 A9 L9 A10
extrude "Extrusion5" add sketch "Sketch2" along normal blind 3 contours A16 L0 | L0 A16 L7 | L7 A23 | A20 L6 L1 | L1 A20 | A22 L6 | A18 L2 | L2 A18 L8 | L8 A21
ref_plane "Work Plane1" through (0, 1.5, 0) normal (0, 1, 0) x (-1, 0, 0)
sketch "Sketch4" plane through (0, 1.5, 0) normal (0, 1, 0) x (-1, 0, 0)
  line L0 (-5.0545, -16.0917) -> (-5.0545, -27.1342) projected
  line L1 (4.9996, -16.0917) -> (4.9996, -27.1342) projected
  line L2 (-5.0545, -18.2625) -> (4.9996, -18.2625)
  line L3 (4.9996, -18.2625) -> (4.9996, -24.8691)
  line L4 (4.9996, -24.8691) -> (-5.0545, -24.8691)
  line L5 (-5.0545, -24.8691) -> (-5.0545, -18.2625)
  point P0 (0, 0)
  constraints: 8 end point, 2 parallel, 2 point on line, 1 horizontal, 1 perpendicular
extrude "Extrusion6" cut sketch "Sketch4" along normal blind 5
fillet "Fillet1" radius 2 2 edges at (-4.9996, 5, -21.7665) (5.0545, 5, -21.756)